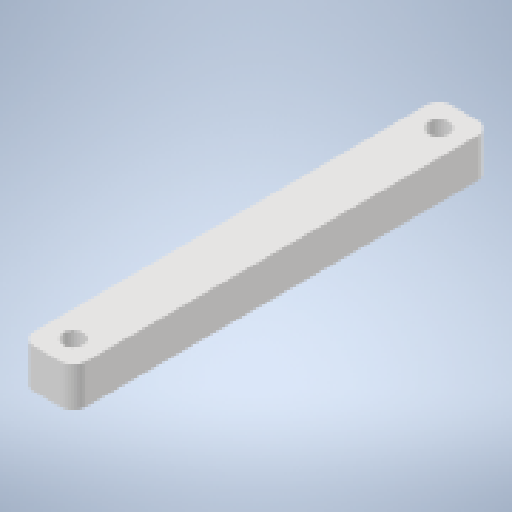
# Autodesk Inventor part: Pusher
Saved by Autodesk Inventor 2023 (Build 270158000, 158)
## iProperties
Created: 2023-02-27
Part Number: Pusher
Material: Generic
Document SubType Name: Modeling
Designer: Gabriel - T3 CAD
Density: 1 g/cm^3
Appearance: Default
Author: Gabriel - T3 CAD
Autodesk Inventor part; units mm, degrees
ref_plane "YZ Plane" through (0, 0, 0) normal (1, 0, 0) x (0, 1, 0)
ref_plane "XZ Plane" through (0, 0, 0) normal (0, 1, 0) x (-1, 0, 0)
ref_plane "XY Plane" through (0, 0, 0) normal (0, 0, 1) x (1, 0, 0)
sketch "Sketch1" plane through (0, 0, 0) normal (0, 1, 0) x (-1, 0, 0)
  line L0 (3.175, 0) -> (9.525, 0)
  line L1 (12.7, 3.175) -> (12.7, 98.425)
  line L2 (9.525, 101.6) -> (3.175, 101.6)
  line L3 (0, 98.425) -> (0, 3.175)
  circle A0 centre (6.35, 95.25) radius 2.5797
  circle A1 centre (6.35, 6.35) radius 2.5797
  arc A2 (12.7, 98.425) -> (9.525, 101.6) centre (9.525, 98.425) ccw
  arc A3 (3.175, 101.6) -> (0, 98.425) centre (3.175, 98.425) ccw
  arc A4 (0, 3.175) -> (3.175, 0) centre (3.175, 3.175) ccw
  arc A5 (9.525, 0) -> (12.7, 3.175) centre (9.525, 3.175) ccw
  point P0 (0, 0)
  point P1 (12.7, 101.6)
  point P2 (0, 101.6)
  dimension "d0" = 12.7
  dimension "d1" = 101.6
  dimension "d2" = 6.35
  dimension "d3" = 6.35
  dimension "d4" = 6.35
  dimension "d5" = 6.35
  dimension "d6" = 5.1594
  dimension "d7" = 3.175
  constraints: 8 end point, 8 point on circle, 8 tangent, 6 centre point, 6 point on line, 4 equal radius, 2 parallel, 1 horizontal, 1 perpendicular
  measures "d0" distance of point (0, 101.6) point (12.7, 101.6)
  measures "d1" distance of point (0, 101.6) point (0, 0)
  measures "d2" distance from line of A1.centre L0
  measures "d3" distance from line of L3 A1.centre
  measures "d4" distance from line of L3 A0.centre
  measures "d5" distance from line of L2 A0.centre
  measures "d6" diameter of A0
  measures "d7" radius of A2
extrude "Extrusion1" add sketch "Sketch1" along normal blind 9.525
equation "\"d2\" = 0.5 * d0"
equation "\"d3\" = d2"
equation "\"d4\" = d3"
equation "\"d5\" = d4"
body "Solid1"
